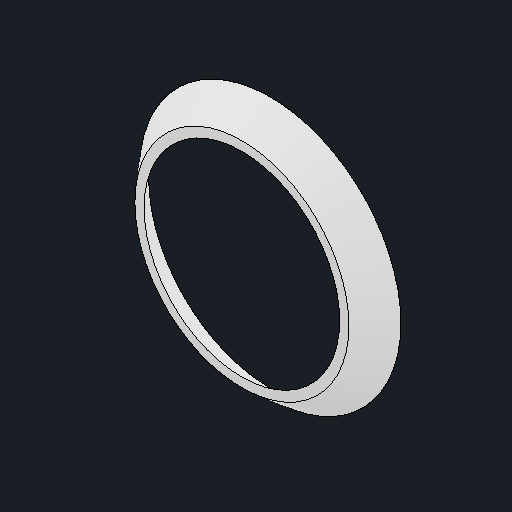
# Autodesk Inventor part: test-internal-cone-overhang
Saved by Autodesk Inventor 2026 (Build 300175050, 175E)
## iProperties
Created: 2026-01-09
Part Number: test-internal-cone-overhang
Material: ABS Plastic
Document SubType Name: Modeling
Designer: kuzmin
Density: 1.06 g/cm^3
Appearance: Smooth - White
Author: kuzmin
Autodesk Inventor part; units mm, degrees
ref_plane "YZ Plane" through (0, 0, 0) normal (1, 0, 0) x (0, 1, 0)
ref_plane "XZ Plane" through (0, 0, 0) normal (0, 1, 0) x (-1, 0, 0)
ref_plane "XY Plane" through (0, 0, 0) normal (0, 0, 1) x (1, 0, 0)
sketch "Sketch1" plane through (0, 0, 0) normal (0, 1, 0) x (-1, 0, 0)
  line L0 (0, 0) -> (0, 20)
  line L1 (0, 20) -> (-75.718, 20)
  line L2 (-75.718, 20) -> (-92.5, 0)
  line L3 (-92.5, 0) -> (0, 0)
  dimension "d0" = 185
  dimension "d1" = 40
  dimension "d2" = 20
  constraints: 8 end point, 1 parallel, 1 perpendicular, 1 vertical
  measures "d0" diameter of L2.end L0
  measures "d1" angle of L0 L2
  measures "d2" distance of L0.start L0.end
revolve "Revolution1" add sketch "Sketch1" angle 360 about axis through (0, 0, 0) along (0, 0, 1)
shell "Shell1" thickness 5 removed faces 2 at (29.4224, 22.5188, 0) at (-17.9688, 19.8766, 20)
equation "\"d1\" = angle"
equation "\"angle\" = 40deg"
body "Solid1"
